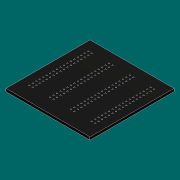
# Autodesk Inventor part: headderPanel
Saved by Autodesk Inventor 2016 SP1 (Build 200210100, 210)
## iProperties
Created: 2015-12-22
Part Number: headderPanel
Material: Generic
Document SubType Name: Modeling
Designer: sawai
Density: 1 g/cm^3
Appearance: Glossy - Black
Author: sawai
Autodesk Inventor part; units mm, degrees
ref_plane "YZ Plane" through (0, 0, 0) normal (1, 0, 0) x (0, 1, 0)
ref_plane "XZ Plane" through (0, 0, 0) normal (0, 1, 0) x (-1, 0, 0)
ref_plane "XY Plane" through (0, 0, 0) normal (0, 0, 1) x (1, 0, 0)
sketch "Sketch1" plane through (0, 0, 0) normal (0, 0, 1) x (1, 0, 0)
  line L0 (-24.25, 24.25) -> (24.25, 24.25)
  line L1 (24.25, 24.25) -> (24.25, -24.25)
  line L2 (24.25, -24.25) -> (-24.25, -24.25)
  line L3 (-24.25, -24.25) -> (-24.25, 24.25)
  line L4 (-24.25, 24.25) -> (24.25, -24.25) construction
  line L5 (24.25, 24.25) -> (-24.25, -24.25) construction
  point P0 (0, 0)
  dimension "d0" = 48.5
  dimension "d1" = 48.5
  constraints: 12 end point, 2 midpoint, 2 parallel, 1 horizontal, 1 perpendicular
  measures "d0" distance of L0.start L0.end
  measures "d1" distance of L0.end L1.end
extrude "Extrusion1" add sketch "Sketch1" along normal blind 1.6
sketch "Sketch2" plane through (0, 0, 1.6) normal (0, 0, 1) x (1, 0, 0)
  line L0 (-19, -18) -> (-17, -18)
  line L1 (-17, -18) -> (-17, 18)
  line L2 (-17, 18) -> (-19, 18)
  line L3 (-19, 18) -> (-19, -18)
  line L4 (-19, -18) -> (-17, 18) construction
  line L5 (-17, -18) -> (-19, 18) construction
  line L6 (0, 0) -> (-18, 0)
  line L7 (-18, 18) -> (-18, -18)
  dimension "d4" = 2
  dimension "d5" = 36
  dimension "d6" = 18
  constraints: 16 end point, 4 midpoint, 2 horizontal, 2 parallel, 1 coincident, 1 perpendicular
  measures "d4" distance of L1.end L2.end
  measures "d5" distance between parallel lines of L2 L0
  measures "d6" distance from line of L6.start L7
hole "Hole1" at (-19, 18, 1.6) direction (0, 0, -1) diameter 0.7071 end through all
pattern_linear "Rectangular Pattern1" count 2 spacing 2 along (1, 0, 0) count 18 spacing 2 along (0, -1, 0) of "Hole1"
pattern_linear "Rectangular Pattern2" count 4 spacing 12 along (1, 0, 0) of "Hole1", "Rectangular Pattern1"
body "Solid1"
